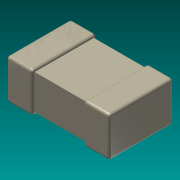
# Autodesk Inventor part: C0805C102K5RACTU
Saved by Autodesk Inventor 2015 (Build 190159000, 159)
## iProperties
Created: 2014-10-16
Part Number: C0805C102K5RACTU
Material: Generic
Document SubType Name: Modeling
Designer: Sawaiz Syed
Density: 1 g/cm^3
Appearance: Light Beige
Author: Sawaiz Syed
Autodesk Inventor part; units mm, degrees
ref_plane "YZ Plane" through (0, 0, 0) normal (1, 0, 0) x (0, 1, 0)
ref_plane "XZ Plane" through (0, 0, 0) normal (0, 1, 0) x (-1, 0, 0)
ref_plane "XY Plane" through (0, 0, 0) normal (0, 0, 1) x (1, 0, 0)
sketch "Sketch1" plane through (0, 0, 0) normal (0, 0, 1) x (1, 0, 0)
  line L0 (1, 0.625) -> (-1, 0.625)
  line L1 (-1, 0.625) -> (-1, -0.625)
  line L2 (-1, -0.625) -> (1, -0.625)
  line L3 (1, -0.625) -> (1, 0.625)
  line L4 (1, 0.625) -> (-1, -0.625) construction
  line L5 (-1, 0.625) -> (1, -0.625) construction
  point P0 (0, 0)
  dimension "d0" = 2
  dimension "d1" = 1.25
  constraints: 12 end point, 2 midpoint, 2 parallel, 1 horizontal, 1 perpendicular
  measures "d0" distance of L2.end L1.end
  measures "d1" distance of L1.end L0.end
sketch "Sketch1 outline for Extrusion1" plane through (0, 0, 0) normal (0, 0, 1) x (1, 0, 0)
  line L0 (1, -0.625) -> (1, 0.625)
  line L1 (-1, -0.625) -> (1, -0.625)
  line L2 (-1, 0.625) -> (-1, -0.625)
  line L3 (1, 0.625) -> (-1, 0.625)
extrude "Extrusion1" add sketch "Sketch1 outline for Extrusion1" along normal mid plane 0.78
sketch "Sketch2" plane through (0, 0, 0.39) normal (0, 0, 1) x (-1, 0, 0)
  line L0 (0.5, 0.624281) -> (0.5, -0.625)
  line L1 (-0.5, 0.625) -> (-0.5, -0.625)
  line L2 (-0.5, 0.625) -> (0.5, 0.625)
  line L3 (0.5, 0.625) -> (0.5, -0.625)
  line L4 (0.5, -0.625) -> (-0.5, -0.625)
  line L5 (-0.5, -0.625) -> (-0.5, 0.625)
  line L6 (-1, -0.625) -> (1, -0.625)
  line L7 (1, 0.625) -> (-1, 0.625)
  line L8 (1, -0.625) -> (1, 0.625)
  line L9 (-1, 0.625) -> (-1, -0.625)
  point P0 (0, 0)
  dimension "d11" = 0.5
  dimension "d12" = 0.5
  constraints: 12 end point, 2 collinear, 2 parallel, 1 horizontal, 1 perpendicular
  measures "d11" distance between parallel lines of L8 L0
  measures "d12" distance between parallel lines of L9 L1
sketch "Sketch2 outline for Extrusion2" plane through (0, 0, 0.39) normal (0, 0, 1) x (-1, 0, 0)
  line L0 (-0.5, -0.625) -> (0.5, -0.625)
  line L1 (-0.5, 0.625) -> (-0.5, -0.625)
  line L2 (0.5, 0.625) -> (-0.5, 0.625)
  line L3 (0.5, -0.625) -> (0.5, 0.625)
extrude "Extrusion2" cut sketch "Sketch2 outline for Extrusion2" against normal blind 0.05
mirror "Mirror1" about plane through (0, 0, 0) normal (0, 0, 1) of "Extrusion2"
sketch "Sketch3" plane through (1, -0.625, -0.39) normal (0, -1, 0) x (1, 0, 0)
  line L0 (-1.5, 0.73) -> (-0.5, 0.73)
  line L1 (-0.5, 0.73) -> (-0.5, 0.05)
  line L2 (-0.5, 0.05) -> (-1.5, 0.05)
  line L3 (-1.5, 0.05) -> (-1.5, 0.73)
  point P0 (-1, 0.39)
  constraints: 8 end point, 2 parallel, 1 horizontal, 1 perpendicular
sketch "Sketch3 outline for Extrusion3" plane through (1, -0.625, -0.39) normal (0, -1, 0) x (1, 0, 0)
  line L0 (-1.5, 0.73) -> (-0.5, 0.73)
  line L1 (-0.5, 0.73) -> (-0.5, 0.05)
  line L2 (-0.5, 0.05) -> (-1.5, 0.05)
  line L3 (-1.5, 0.05) -> (-1.5, 0.73)
extrude "Extrusion3" cut sketch "Sketch3 outline for Extrusion3" against normal blind 0.05
mirror "Mirror2" about plane through (0, 0, 0) normal (0, 1, 0) of "Extrusion3"
fillet "Fillet1" radius 0.05 24 edges at (0.75, 0.625, 0.39) (1, 0.625, 0) (0.75, 0.625, -0.39) (0.75, -0.625, -0.39) (1, -0.625, 0) (0.75, -0.625, 0.39) (-0.75, -0.625, 0.39) (-1, -0.625, 0) (-0.75, -0.625, -0.39) (1, 0, -0.39) (1, 0, 0.39) (-0.75, 0.625, 0.39) (-1, 0, 0.39) (-0.75, 0.625, -0.39) (-1, 0.625, 0) (-1, 0, -0.39) (-0.5, 0.625, 0) (-0.5, 0, 0.39) (-0.5, -0.625, 0) (-0.5, 0, -0.39) (0.5, 0.625, 0) (0.5, 0, -0.39) (0.5, -0.625, 0) (0.5, 0, 0.39)
body "Solid1"
